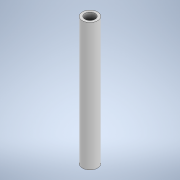
# Autodesk Inventor part: body
Saved by Autodesk Inventor 2022 (Build 260153000, 153)
## iProperties
Created: 2023-01-18
Part Number: body
Material: Generic
Document SubType Name: Modeling
Designer: CLCK
Density: 1 g/cm^3
Appearance: Default
Author: CLCK
Autodesk Inventor part; units mm, degrees
ref_plane "YZ Plane" through (0, 0, 0) normal (1, 0, 0) x (0, 1, 0)
ref_plane "XZ Plane" through (0, 0, 0) normal (0, 1, 0) x (-1, 0, 0)
ref_plane "XY Plane" through (0, 0, 0) normal (0, 0, 1) x (1, 0, 0)
sketch "Sketch2" plane through (0, 0, 0) normal (1, 0, 0) x (0, 1, 0)
  line L0 (50, 4) -> (-50, 4)
  line L1 (-50, 4) -> (-50, -4)
  line L2 (-50, -4) -> (50, -4)
  line L3 (50, -4) -> (50, 4)
  line L4 (50, 4) -> (-50, -4) construction
  line L5 (-50, 4) -> (50, -4) construction
  line L6 (50, 6) -> (-50, 6)
  line L7 (-50, 6) -> (-50, -6)
  line L8 (-50, -6) -> (50, -6)
  line L9 (50, -6) -> (50, 6)
  line L10 (50, 6) -> (-50, -6) construction
  line L11 (-50, 6) -> (50, -6) construction
  line L12 (50, 0) -> (-50, 0)
  point P0 (0, 0)
  dimension "d0" = 100
  dimension "d1" = 8
  dimension "d2" = 100
  dimension "d3" = 12
  constraints: 26 end point, 6 midpoint, 4 parallel, 2 horizontal, 2 perpendicular
  measures "d0" distance of L2.end L1.end
  measures "d1" distance of L1.end L0.end
  measures "d2" distance of L8.end L7.end
  measures "d3" distance of L7.end L6.end
revolve "Revolution1" add sketch "Sketch2" angle 360 about axis through (0, 50, 0) along (0, -1, 0) contours L9 L8 L7 L2
sketch "Sketch3" plane through (0, 0, 0) normal (1, 0, 0) x (0, 1, 0)
  line L0 (-29, 4) -> (-31, 4)
  line L1 (-31, 4) -> (-31, -4)
  line L2 (-31, -4) -> (-29, -4)
  line L3 (-29, -4) -> (-29, 4)
  line L4 (-29, 4) -> (-31, -4) construction
  line L5 (-31, 4) -> (-29, -4) construction
  line L6 (-29, 3) -> (-31, 3)
  line L7 (-31, 3) -> (-31, -3)
  line L8 (-31, -3) -> (-29, -3)
  line L9 (-29, -3) -> (-29, 3)
  line L10 (-29, 3) -> (-31, -3) construction
  line L11 (-31, 3) -> (-29, -3) construction
  line L12 (-30, 0) -> (-57.704, 0)
  line L13 (-50, 4) -> (-50, -4) projected
  point P0 (0, 0)
  dimension "d5" = 2
  dimension "d6" = 8
  dimension "d7" = 2
  dimension "d8" = 6
  constraints: 26 end point, 5 midpoint, 4 parallel, 3 perpendicular, 2 horizontal
  measures "d5" distance of L2.end L1.end
  measures "d6" distance of L1.end L0.end
  measures "d7" distance of L8.end L7.end
  measures "d8" distance of L7.end L6.end
revolve "Revolution2" add sketch "Sketch3" angle 360 about axis through (0, -30, 0) along (0, -1, 0) contours L3 L2 L1 L8
body "Solid1"
